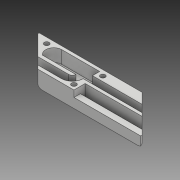
# Autodesk Inventor part: circuitcover
Saved by Autodesk Inventor 2018 (Build 220112000, 112)
## iProperties
Created: 2019-02-21
Part Number: circuitcover
Material: 一般
Document SubType Name: Modeling
Designer: ku_sk
Density: 1 g/cm^3
Appearance: 既定
Author: ku_sk
Autodesk Inventor part; units mm, degrees
ref_plane "YZ Plane" through (0, 0, 0) normal (1, 0, 0) x (0, 1, 0)
ref_plane "XZ Plane" through (0, 0, 0) normal (0, 1, 0) x (-1, 0, 0)
ref_plane "XY Plane" through (0, 0, 0) normal (0, 0, 1) x (1, 0, 0)
sketch "スケッチ1" plane through (0, 0, 0) normal (0, 0, 1) x (1, 0, 0)
  line L0 (-52.5, 20) -> (-32.5, 0)
  line L1 (-32.5, 0) -> (32.5, 0)
  line L2 (32.5, 0) -> (12.5, 20)
  line L3 (12.5, 20) -> (-52.5, 20)
  point P0 (0, 0)
  point P1 (0, 0)
  dimension "d0" = 45
  dimension "d1" = 20
  dimension "d2" = 65
  constraints: 8 end point, 2 parallel, 1 coincident, 1 horizontal, 1 midpoint
  measures "d0" angle of L1 L0
  measures "d1" distance between parallel lines of L1 L3
  measures "d2" distance of L0.end L1.end
extrude "押し出し1" add sketch "スケッチ1" along normal mid plane 20
sketch "スケッチ3" plane through (0, 0, 0) normal (1, 0, 0) x (0, 1, 0)
  line L0 (0, -10) -> (0, 10) projected
  line L1 (0, 4) -> (4, 4)
  line L2 (4, 4) -> (4, 7.75)
  line L3 (4, 7.75) -> (7, 7.75)
  line L4 (7, 7.75) -> (7, -7.75)
  line L5 (7, -7.75) -> (4, -7.75)
  line L6 (4, -7.75) -> (4, -4)
  line L7 (4, -4) -> (0, -4)
  line L8 (0, 4) -> (0, -4)
  line L9 (0, -10) -> (0, 10) projected
  point P0 (0, 0)
  point P1 (0, 0)
  dimension "d15" = 15.5
  dimension "d16" = 3
  dimension "d17" = 4
  dimension "d18" = 3.75
  dimension "d19" = 3.75
  constraints: 16 end point, 6 perpendicular, 4 point on line, 2 midpoint, 1 horizontal
  measures "d15" distance of L3.end L4.end
  measures "d16" distance of L2.end L3.end
  measures "d17" distance of L1.start L1.end
  measures "d18" distance of L1.end L2.end
  measures "d19" distance of L5.end L6.end
extrude "押し出し3" cut sketch "スケッチ3" along normal blind 35 and the other way blind 10
sketch "スケッチ4" plane through (0, 0, 0) normal (0, 0, 1) x (1, 0, 0)
  line L0 (-55.8638, 29.4692) -> (38.5404, 29.4692)
  line L1 (38.5404, 29.4692) -> (38.5404, -5.99)
  line L2 (38.5404, -5.99) -> (-55.8638, -5.99)
  line L3 (-55.8638, -5.99) -> (-55.8638, 29.4692)
  point P0 (0, 0)
  constraints: 8 end point, 2 parallel, 1 horizontal, 1 perpendicular
extrude "押し出し4" cut sketch "スケッチ4" along normal blind 30
shell "シェル1" thickness 2 removed faces 1 at (-16.6667, 15.6667, 0)
fillet "フィレット2" radius 5 1 edges at (-47.6716, 18, -4)
sketch "スケッチ7" plane through (-31.6716, 2, -8) normal (0, 0, 1) x (1, 0, 0)
  arc A0 (-3.9289, 16) -> (-7.4645, 7.4645) centre (-3.9289, 11) ccw projected
  line L0 (0, 0) -> (-7.4645, 7.4645) projected
  line L1 (19.6716, 0) -> (0, 0) projected
  line L2 (19.6716, 0) -> (19.6716, 7) projected
  line L3 (19.6716, 7) -> (52.3431, 7) projected
  line L4 (43.3431, 16) -> (52.3431, 7) projected
  line L5 (-3.9289, 16) -> (43.3431, 16) projected
  line L6 (19.6716, 7) -> (-7, 7)
  line L7 (19.6716, 7) -> (19.7071, 16)
  line L8 (-3.9289, 16) -> (43.3431, 16) projected
  point P0 (31.6716, -2)
  constraints: 4 end point, 1 horizontal, 1 midpoint, 1 point on line
extrude "押し出し6" add sketch "スケッチ7" along normal up to surface (8 mm away) contours L5 L4 L3 L7 | L6 L2 L1 L0
ref_plane "作業平面1" through (32.5, 0, -4) normal (-1, 0, 0) x (0, -1, 0)
sketch "スケッチ8" plane through (32.5, 0, -4) normal (-1, 0, 0) x (0, -1, 0)
  line L0 (-9, 4) -> (-9, -1)
  line L1 (-9, 4) -> (-13.5, 4)
  line L2 (-13.5, 4) -> (-13.5, -1)
  arc A0 (-13.5, -1) -> (-9, -1) centre (-11.25, -1) ccw
  line L3 (-20, 4) -> (-7, 4) projected
  point P0 (0, 4)
  dimension "d42" = 5
  dimension "d43" = 2.25
  constraints: 6 end point, 2 perpendicular, 2 point on circle, 2 tangent, 1 centre point, 1 collinear, 1 vertical
  measures "d42" distance from line of L1 A0.centre
  measures "d43" radius of A0
sketch "スケッチ9" plane through (0, 0, 0) normal (0, 0, 1) x (1, 0, 0)
  line L0 (32.5, 9) -> (32.5, 13.5) projected
  line L1 (32.5, 11.25) -> (-16.1029, 11.25)
  arc A0 (-20, 4.5) -> (-16.1029, 11.25) centre (-20, 9) ccw
  line L2 (-38.6716, 9) -> (-12, 9) projected
  line L3 (-20, 4.5) -> (-37, 4.5)
  line L4 (-32.5, 0) -> (-52.5, 20) projected
  line L5 (-10, 0) -> (-32.5, 0) projected
  point P0 (0, 0)
  point P1 (-47.7255, 15.2255)
  dimension "d44" = 4.5
  dimension "d45" = 17
  constraints: 4 end point, 2 horizontal, 2 point on circle, 1 centre point, 1 line through centre, 1 midpoint, 1 point on line, 1 tangent
  measures "d44" distance between parallel lines of L5 L3
  measures "d45" distance of L3.start L3.end
sweep "スイープ1" cut profiles "スケッチ8" path "スケッチ9" path curves L1 A0 L3
sketch "スケッチ10" plane through (-37, 4.5, 0) normal (1, 0, 0) x (0, 0, -1)
  line L0 (7.25, 0) -> (0, 0) projected
  arc A0 (7.25, 0) -> (5, 2.25) centre (5, 0) ccw projected
  line L1 (0, 2.25) -> (5, 2.25) projected
  line L2 (0, 0) -> (0, 2.25) projected
  point P0 (0, -4.5)
extrude "押し出し7" cut sketch "スケッチ10" against normal blind 30
sketch "スケッチ6" plane through (0, 0, 0) normal (0, 0, 1) x (1, 0, 0)
  circle A0 centre (-43.5, 16.5) radius 1.5
  line L0 (-52.5, 20) -> (12.5, 20) projected
  circle A1 centre (-8.5, 16.5) radius 1.5
  circle A2 centre (-13, 3) radius 1.5
  line L1 (-10, 7) -> (-10, 0) projected
  line L2 (-10, 0) -> (-32.5, 0) projected
  point P0 (0, 0)
  point P1 (-47.7255, 20)
  dimension "d34" = 3.5
  dimension "d35" = 9
  dimension "d36" = 3
  dimension "d37" = 35
  dimension "d38" = 3.5
  dimension "d39" = 3
  dimension "d50" = 3
  dimension "d51" = 3
  dimension "d52" = 3
  constraints: 3 centre point
  measures "d34" distance from line of L0 A0.centre
  measures "d35" horizontal distance of L0.start A0.centre
  measures "d36" diameter of A0
  measures "d37" distance of A0.centre A1.centre
  measures "d38" distance from line of L0 A1.centre
  measures "d39" diameter of A1
  measures "d50" diameter of A2
  measures "d51" distance from line of L1 A2.centre
  measures "d52" distance from line of L2 A2.centre
extrude "押し出し8" cut sketch "スケッチ6" against normal blind 30
chamfer "面取り1" distance 1 angle 45 2 edges at (-52.5, 20, -5) (32.5, 0, -7)
fillet "フィレット4" radius 2 3 edges at (-42.1464, 9.6464, -10) (-19.5, 20, -10) (22.1464, 10.3536, -10)
equation "\"d19\" = d18"
equation "\"d50\" = d39"
